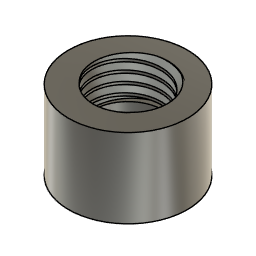
Thread Test Nut (Autodesk Fusion 360 design; units mm, degrees)
Autodesk Fusion 360 part; units mm, degrees
sketch "Sketch1" plane through (0, 0, 0) normal (0, 0, 1) x (1, 0, 0)
  circle A0 centre (0, 0) radius 15
  circle A1 centre (0, 0) radius 10
  dimension "d1" = 30
  constraint coincident A0.centre A1.centre
  constraint concentric A0 A1
  measures "d1" diameter of A0
extrude "Extrude1" add sketch "Sketch1" along normal blind 20
thread "Thread1" "ISO Metric profile 20.0 M20x2.5 6H" major diameter 20.2925 minor diameter 17.519 pitch 2.5 angle 60 modelled right hand crest width 0.6905 on face at (9.9876, -0.4985, 13.3333) from (0, 0, 10) to (0, 0, 20) crest through (8.7595, 0, 0.625)
